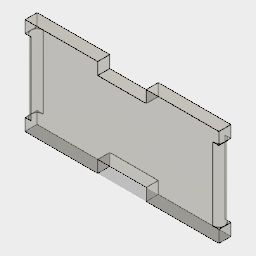
Top frame mount (Autodesk Fusion 360 design; units mm, degrees)
Autodesk Fusion 360 part; units mm, degrees
note: some values were not read from the file. Chosen so that the rebuilt part matches the saved one: which bodies a step acts on.
sketch "Sketch1" plane through (0, 0, 0) normal (0, 0, 1) x (1, 0, 0)
  line L0 (0, 0) -> (203.2, 0)
  line L1 (203.2, 0) -> (203.2, 76.2)
  line L2 (203.2, 76.2) -> (0, 76.2)
  line L3 (0, 76.2) -> (0, 0)
  line L4 (0, 76.2) -> (0, 88.9)
  line L5 (0, 88.9) -> (76.2, 88.9)
  line L6 (76.2, 88.9) -> (76.2, 76.2)
  line L7 (203.2, 76.2) -> (203.2, 88.9)
  line L8 (203.2, 88.9) -> (127, 88.9)
  line L9 (127, 88.9) -> (127, 76.2)
  line L10 (0, 38.1) -> (203.2, 38.1)
  line L11 (203.2, 0) -> (203.2, -12.7)
  line L12 (203.2, -12.7) -> (127, -12.7)
  line L13 (127, -12.7) -> (127, 0)
  line L14 (76.2, -12.7) -> (76.2, 0)
  line L15 (0, -12.7) -> (76.2, -12.7)
  line L16 (0, 0) -> (0, -12.7)
  dimension "d1" = 203.2
  dimension "d2" = 76.2
  dimension "d7" = 12.7
  dimension "d8" = 76.2
  dimension "d9" = 12.7
  dimension "d10" = 76.2
  measures "d1" distance of L0.start L0.end
  measures "d2" distance of L0.start L2.end
  measures "d7" distance of L2.end L4.end
  measures "d8" distance of L4.end L5.end
  measures "d9" distance of L1.end L7.end
  measures "d10" distance of L7.end L8.end
extrude "Extrude1" add sketch "Sketch1" along normal blind 12.7 contours L0 L1 L3 L10 | L1 L2 L3 L10 makes body 1
extrude "Extrude2" add sketch "Sketch1" along normal blind 12.7 contours L0 L14 L15 L16 | L0 L11 L12 L13 | L2 L4 L5 L6 | L2 L7 L8 L9 bodies 1
split "Split1" by plane through (0, 0, 0) normal (0, 1, 0) bodies 1 makes body 2 at (177.8, -4.2333, 0) makes body 3 at (25.4, 55.0333, 0)
split "Split2" by plane through (203.2, 76.2, 0) normal (0, 1, 0) bodies 3 makes body 4 at (50.8, 80.4333, 0) makes body 5 at (177.8, 80.4333, 0)
fillet "Fillet3" radius 6.35 2 edges at (203.2, 38.1, 12.7) (203.2, 38.1, 0) on bodies 3
fillet "Fillet4" radius 6.35 2 edges at (0, 38.1, 0) (0, 38.1, 12.7) on bodies 3
combine "Combine1" operation add target body 3 tool bodies 4 5 2 1
